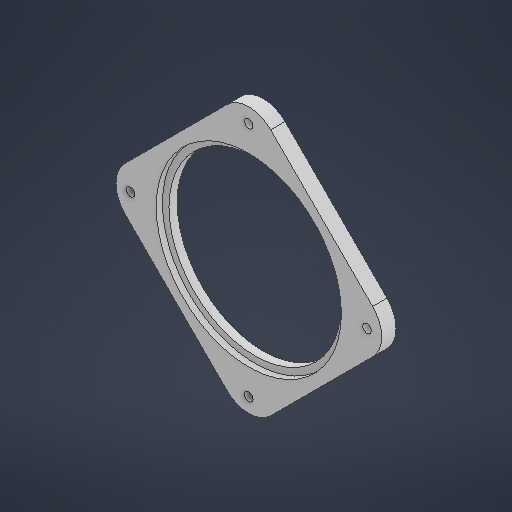
# Autodesk Inventor part: Fix_bearing_Base
Saved by Autodesk Inventor 2025.2 (Build 292293000, 293)
## iProperties
Created: 2025-07-10
Part Number: Fix_bearing_Base
Material: Generic
Document SubType Name: Modeling
Designer: Tiago
Density: 1 g/cm^3
Appearance: Default
Author: Tiago
Autodesk Inventor part; units mm, degrees
ref_plane "YZ Plane" through (0, 0, 0) normal (1, 0, 0) x (0, 1, 0)
ref_plane "XZ Plane" through (0, 0, 0) normal (0, 1, 0) x (-1, 0, 0)
ref_plane "XY Plane" through (0, 0, 0) normal (0, 0, 1) x (1, 0, 0)
sketch "Sketch1" plane through (0, 0, 0) normal (0, 0, 1) x (1, 0, 0)
  circle A0 centre (0, 0) radius 44.925
  circle A1 centre (0, 0) radius 57.417 construction
  circle A2 centre (-57.417, 0) radius 2.1
  circle A3 centre (0, -57.417) radius 2.1
  circle A4 centre (57.417, 0) radius 2.1
  circle A5 centre (0, 57.417) radius 2.1
  circle A6 centre (0, 0) radius 41.75
  line L0 (0, 62.3245) -> (4.25, 59.8707)
  line L1 (4.25, 59.8707) -> (4.25, 54.9633)
  line L2 (4.25, 54.9633) -> (0, 52.5095)
  line L3 (0, 52.5095) -> (-4.25, 54.9633)
  line L4 (-4.25, 54.9633) -> (-4.25, 59.8707)
  line L5 (-4.25, 59.8707) -> (0, 62.3245)
  line L6 (60.1041, 10.6066) -> (10.6066, 60.1041)
  line L7 (-10.6066, 60.1041) -> (-60.1041, 10.6066)
  line L8 (-60.1041, -10.6066) -> (-10.6066, -60.1041)
  line L9 (10.6066, -60.1041) -> (60.1041, -10.6066)
  arc A7 (-10.6066, -60.1041) -> (10.6066, -60.1041) centre (0, -49.4975) ccw
  arc A8 (-60.1041, 10.6066) -> (-60.1041, -10.6066) centre (-49.4975, 0) ccw
  arc A9 (10.6066, 60.1041) -> (-10.6066, 60.1041) centre (0, 49.4975) ccw
  arc A10 (60.1041, -10.6066) -> (60.1041, 10.6066) centre (49.4975, 0) ccw
  line L10 (-59.8707, -4.25) -> (-62.3245, 0)
  line L11 (-54.9633, -4.25) -> (-59.8707, -4.25)
  line L12 (-62.3245, 0) -> (-59.8707, 4.25)
  line L13 (-59.8707, 4.25) -> (-54.9633, 4.25)
  line L14 (-54.9633, 4.25) -> (-52.5095, 0)
  line L15 (-52.5095, 0) -> (-54.9633, -4.25)
  line L16 (4.25, -59.8707) -> (0, -62.3245)
  line L17 (4.25, -54.9633) -> (4.25, -59.8707)
  line L18 (0, -62.3245) -> (-4.25, -59.8707)
  line L19 (-4.25, -59.8707) -> (-4.25, -54.9633)
  line L20 (-4.25, -54.9633) -> (0, -52.5095)
  line L21 (0, -52.5095) -> (4.25, -54.9633)
  line L22 (59.8707, 4.25) -> (62.3245, 0)
  line L23 (54.9633, 4.25) -> (59.8707, 4.25)
  line L24 (62.3245, 0) -> (59.8707, -4.25)
  line L25 (59.8707, -4.25) -> (54.9633, -4.25)
  line L26 (54.9633, -4.25) -> (52.5095, 0)
  line L27 (52.5095, 0) -> (54.9633, 4.25)
  point P0 (70.7107, 0)
  point P1 (0, 70.7107)
  point P2 (-70.7107, 0)
  point P3 (0, -70.7107)
  dimension "d1" = 114.834
  dimension "d0" = 89.85
  dimension "d2" = 4.2
  dimension "d5" = 360
  dimension "d8" = 83.5
  dimension "d18" = 8.5
  dimension "d25" = 100
  dimension "d26" = 100
  dimension "d27" = 15
  dimension "d30" = 360
  constraints: 56 end point, 10 centre point, 8 point on circle, 8 point on line, 8 tangent, 4 coincident, 3 equal radius, 3 horizontal alignment, 3 vertical alignment, 2 parallel, 1 perpendicular, 73 other
  measures "d0" diameter of A0
  measures "d2" diameter of A2
  measures "d8" diameter of A6
  measures "d18" distance between parallel lines of L1 L4
  measures "d25" distance of point (0, 70.711) point (-70.711, 0)
  measures "d26" distance of point (-70.711, 0) point (0, -70.711)
  measures "d27" radius of A7
extrude "Extrusion1" add sketch "Sketch1" along normal blind 7 contours L0 L1 L2 L3 L4 L5 | A10 L9 A7 L8 A8 L7 A9 L6 | L10 L12 L13 L14 L15 L11 | L16 L18 L19 L20 L21 L17 | L22 L24 L25 L26 L27 L23
extrude "Extrusion2" add sketch "Sketch1" along normal blind 4 contours A0
extrude "Extrusion3" cut sketch "Sketch1" along normal blind 4 contours A2 | A3 | A4 | A5 | L0 L1 L2 L3 L4 L5 | L10 L12 L13 L14 L15 L11 | L16 L18 L19 L20 L21 L17 | L22 L24 L25 L26 L27 L23
body "Solid1"
